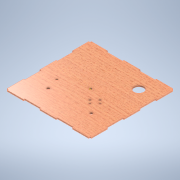
# Autodesk Inventor part: FloorPlateBottom_V2
Saved by Autodesk Inventor 2022.2 (Build 262287000, 287)
## iProperties
Created: 2022-11-22
Part Number: FloorPlateBottom_V2
Material: Wood (Oak)
Document SubType Name: Modeling
Designer: jaege
Density: 0.76 g/cm^3
Appearance: Red Oak - Natural Low Gloss
Mass: 194.404 g
Surface Area: 1333.29 cm^2
Volume: 255.795 cm^3
Author: jaege
Autodesk Inventor part; units mm, degrees
ref_plane "YZ Plane" through (0, 0, 0) normal (1, 0, 0) x (0, 1, 0)
ref_plane "XZ Plane" through (0, 0, 0) normal (0, 1, 0) x (-1, 0, 0)
ref_plane "XY Plane" through (0, 0, 0) normal (0, 0, 1) x (1, 0, 0)
sketch "Sketch1" plane through (0, 0, 0) normal (0, 1, 0) x (-1, 0, 0)
  line L0 (-125, 125) -> (125, 125)
  line L1 (125, 125) -> (125, -125)
  line L2 (125, -125) -> (-125, -125)
  line L3 (-125, -125) -> (-125, 125)
  line L4 (-125, 125) -> (125, -125) construction
  line L5 (125, 125) -> (-125, -125) construction
  line L6 (125, -125) -> (75, -125)
  line L7 (75, -125) -> (75, -129)
  line L8 (75, -129) -> (125, -129)
  line L9 (125, -129) -> (125, -125)
  line L10 (125, -125) -> (129, -125)
  line L11 (129, -125) -> (129, -75)
  line L12 (129, -75) -> (125, -75)
  line L13 (125, -75) -> (125, -125)
  line L14 (-125, -125) -> (-129, -125)
  line L15 (-129, -125) -> (-129, -75)
  line L16 (-129, -75) -> (-125, -75)
  line L17 (-125, -75) -> (-125, -125)
  line L18 (125, 125) -> (75, 125)
  line L19 (75, 125) -> (75, 129)
  line L20 (75, 129) -> (125, 129)
  line L21 (125, 129) -> (125, 125)
  line L22 (75, -129) -> (75, -125)
  line L23 (75, -125) -> (25, -125)
  line L24 (25, -125) -> (25, -129)
  line L25 (25, -129) -> (75, -129)
  line L26 (25, -129) -> (25, -125)
  line L27 (25, -125) -> (-25, -125)
  line L28 (-25, -125) -> (-25, -129)
  line L29 (-25, -129) -> (25, -129)
  line L30 (-25, -129) -> (-25, -125)
  line L31 (-25, -125) -> (-75, -125)
  line L32 (-75, -125) -> (-75, -129)
  line L33 (-75, -129) -> (-25, -129)
  line L34 (-75, -129) -> (-75, -125)
  line L35 (-75, -125) -> (-125, -125)
  line L36 (-125, -125) -> (-125, -129)
  line L37 (-125, -129) -> (-75, -129)
  line L38 (125, -75) -> (129, -75)
  line L39 (125, -25) -> (125, -75)
  line L40 (129, -25) -> (125, -25)
  line L41 (129, -75) -> (129, -25)
  line L42 (125, -25) -> (129, -25)
  line L43 (125, 25) -> (125, -25)
  line L44 (129, 25) -> (125, 25)
  line L45 (129, -25) -> (129, 25)
  line L46 (125, 25) -> (129, 25)
  line L47 (125, 75) -> (125, 25)
  line L48 (129, 75) -> (125, 75)
  line L49 (129, 25) -> (129, 75)
  line L50 (125, 75) -> (129, 75)
  line L51 (125, 125) -> (125, 75)
  line L52 (129, 125) -> (125, 125)
  line L53 (129, 75) -> (129, 125)
  line L54 (-125, -75) -> (-129, -75)
  line L55 (-129, -75) -> (-129, -25)
  line L56 (-129, -25) -> (-125, -25)
  line L57 (-125, -25) -> (-125, -75)
  line L58 (-125, -25) -> (-129, -25)
  line L59 (-129, -25) -> (-129, 25)
  line L60 (-129, 25) -> (-125, 25)
  line L61 (-125, 25) -> (-125, -25)
  line L62 (-125, 25) -> (-129, 25)
  line L63 (-129, 25) -> (-129, 75)
  line L64 (-129, 75) -> (-125, 75)
  line L65 (-125, 75) -> (-125, 25)
  line L66 (-125, 75) -> (-129, 75)
  line L67 (-129, 75) -> (-129, 125)
  line L68 (-129, 125) -> (-125, 125)
  line L69 (-125, 125) -> (-125, 75)
  line L70 (75, 125) -> (25, 125)
  line L71 (25, 125) -> (25, 129)
  line L72 (25, 129) -> (75, 129)
  line L73 (75, 129) -> (75, 125)
  line L74 (25, 125) -> (-25, 125)
  line L75 (-25, 125) -> (-25, 129)
  line L76 (-25, 129) -> (25, 129)
  line L77 (25, 129) -> (25, 125)
  line L78 (-25, 125) -> (-75, 125)
  line L79 (-75, 125) -> (-75, 129)
  line L80 (-75, 129) -> (-25, 129)
  line L81 (-25, 129) -> (-25, 125)
  line L82 (-75, 125) -> (-125, 125)
  line L83 (-125, 125) -> (-125, 129)
  line L84 (-125, 129) -> (-75, 129)
  line L85 (-75, 129) -> (-75, 125)
  point P0 (0, 0)
  dimension "d0" = 250
  dimension "d1" = 250
  dimension "d2" = 50
  dimension "d3" = 4
  dimension "d4" = 4
  dimension "d5" = 50
  dimension "d6" = 4
  dimension "d7" = 50
  dimension "d8" = 50
  dimension "d9" = 4
  dimension "d12" = 50
  dimension "d19" = 50
  dimension "d26" = 50
  dimension "d33" = 50
  constraints: 172 end point, 10 parallel, 7 horizontal, 5 perpendicular, 2 midpoint, 2 vertical, 136 other
  measures "d0" distance of L1.end L2.end
  measures "d1" distance of L0.end L1.end
  measures "d2" distance of L8.end L7.end
  measures "d3" distance of L7.end L6.end
  measures "d4" distance of L12.end L11.end
  measures "d5" distance of L11.end L10.end
  measures "d6" distance of L15.end L16.end
  measures "d7" distance of L14.end L15.end
  measures "d8" distance of L19.end L20.end
  measures "d9" distance of L18.end L19.end
  measures "d12" distance of L1.end L22.end
  measures "d19" distance of L1.end L38.start
  measures "d26" distance of L2.end L54.start
  measures "d33" distance of L0.end L70.start
extrude "Extrusion1" add sketch "Sketch1" along normal blind 4 contours L83 L84 L79 L0 | L0 L1 L2 L3 | L3 L64 L67 L68 | L75 L76 L71 L0 | L3 L56 L59 L60 | L19 L20 L21 L0 | L3 L14 L15 L16 | L52 L53 L48 L1 | L2 L32 L37 L36 | L44 L45 L40 L1 | L2 L24 L29 L28 | L12 L11 L10 L1 | L2 L9 L8 L7
sketch "Sketch2" plane through (0, 4, 0) normal (0, 1, 0) x (1, 0, 0)
  line L0 (25, -125) -> (75, -125) construction
  circle A0 centre (0, 2.3) radius 3.5
  line L1 (-8.45, 2.3) -> (8.45, 2.3) construction
  line L2 (-8.45, 1.0705) -> (8.45, 1.0705) construction
  line L3 (8.45, 3.5295) -> (-8.45, 3.5295) construction
  arc A1 (-8.45, 3.5295) -> (-8.45, 1.0705) centre (-8.45, 2.3) ccw construction
  arc A2 (8.45, 1.0705) -> (8.45, 3.5295) centre (8.45, 2.3) ccw construction
  circle A3 centre (8.45, 2.3) radius 1.2295
  circle A4 centre (-8.45, 2.3) radius 1.2295
  circle A5 centre (-66, -62.2) radius 4
  circle A6 centre (66, -62.2) radius 4
  line L4 (0, 180.6) -> (0, -180.6) construction
  line L5 (-93.2324, -124) -> (95.467, -124) construction
  line L6 (-129, -125) -> (-125, -125) projected
  line L7 (25, -29.4721) -> (29.2426, -25.2294)
  line L8 (44.799, -9.6731) -> (47.6274, -12.5015)
  line L9 (47.6274, -12.5015) -> (43.3848, -16.7442)
  line L10 (27.8284, -32.3005) -> (25, -29.4721)
  line L11 (34.8995, -39.3716) -> (39.1421, -35.1289)
  line L12 (54.6985, -19.5726) -> (57.5269, -22.401)
  line L13 (57.5269, -22.401) -> (53.2843, -26.6437)
  line L14 (37.7279, -42.2) -> (34.8995, -39.3716)
  line L15 (40.5563, -13.9157) -> (43.3848, -16.7442)
  line L16 (29.2426, -25.2294) -> (32.0711, -28.0579)
  line L17 (39.1421, -35.1289) -> (41.9706, -37.9574)
  line L18 (50.4558, -23.8152) -> (53.2843, -26.6437)
  line L19 (40.5563, -13.9157) -> (44.799, -9.6731)
  line L20 (29.2426, -25.2294) -> (40.5563, -13.9157) construction
  line L21 (43.3848, -16.7442) -> (32.0711, -28.0579) construction
  line L22 (50.4558, -23.8152) -> (54.6985, -19.5726)
  line L23 (53.2843, -26.6437) -> (41.9706, -37.9574) construction
  line L24 (32.0711, -28.0579) -> (27.8284, -32.3005)
  line L25 (39.1421, -35.1289) -> (50.4558, -23.8152) construction
  line L26 (41.9706, -37.9574) -> (37.7279, -42.2)
  point P0 (0, 0)
  point P1 (26.4142, -30.8863)
  dimension "d46" = 7
  dimension "d47" = 16.9
  dimension "d48" = 1.2295
  dimension "d52" = 8
  dimension "d53" = 132
  dimension "d54" = 61.8
  dimension "d55" = 1
  dimension "d56" = 64.5
  dimension "d57" = 10
  dimension "d58" = 4
  dimension "d59" = 6
  dimension "d60" = 6
  dimension "d61" = 45
  dimension "d62" = 20
  dimension "d63" = 28
  dimension "d64" = 25
  constraints: 50 end point, 21 parallel, 15 perpendicular, 7 centre point, 6 point on line, 4 point on circle, 4 tangent, 3 collinear, 3 equal radius, 2 coincident, 2 horizontal, 2 midpoint, 1 horizontal alignment, 1 symmetric about line, 1 vertical alignment
  measures "d46" diameter of A0
  measures "d47" distance of L1.start L1.end
  measures "d48" radius of A2
  measures "d52" diameter of A5
  measures "d53" distance of A6.centre A5.centre
  measures "d54" distance from line of A6.centre L5
  measures "d55" distance between parallel lines of L6 L5
  measures "d56" vertical distance of A5.centre A0.centre
  measures "d57" distance between parallel lines of L11 L9
  measures "d58" distance of L8.start L8.end
  measures "d59" distance of L8.start L15.start
  measures "d60" distance from line of point (26.414, -30.886) L16
  measures "d61" angle of L4 L7
  measures "d62" vertical distance of A6.centre L14.start
  measures "d63" distance of L12.end L14.start
  measures "d64" distance from line of L4 L7.start
extrude "Extrusion2" cut sketch "Sketch2" against normal up to next
sketch "Sketch3" plane through (0, 4, 0) normal (0, 1, 0) x (1, 0, 0)
  point P0 (0, 0)
sketch "Sketch4" plane through (0, 4, 0) normal (0, 1, 0) x (1, 0, 0)
  circle A0 centre (75, 75) radius 15
  line L0 (125, 25) -> (125, 75) projected
  line L1 (75, 125) -> (25, 125) projected
  point P0 (0, 0)
  dimension "d65" = 30
  dimension "d66" = 50
  dimension "d67" = 50
  constraints: 1 centre point
  measures "d65" diameter of A0
  measures "d66" distance from line of L0 A0.centre
  measures "d67" distance from line of L1 A0.centre
extrude "Extrusion3" cut sketch "Sketch4" against normal through all
sketch "Sketch5" plane through (0, 4, 0) normal (0, 1, 0) x (1, 0, 0)
  circle A0 centre (75, 75) radius 15 projected
  line L0 (54.6985, -19.5726) -> (57.5269, -22.401) projected
  line L1 (57.5269, -22.401) -> (53.2843, -26.6437) projected
  line L2 (53.2843, -26.6437) -> (50.4558, -23.8152) projected
  line L3 (50.4558, -23.8152) -> (54.6985, -19.5726) projected
  circle A1 centre (8.45, 2.3) radius 1.2295 projected
  circle A2 centre (0, 2.3) radius 3.5 projected
  line L4 (39.1421, -35.1289) -> (41.9706, -37.9574) projected
  line L5 (41.9706, -37.9574) -> (37.7279, -42.2) projected
  line L6 (37.7279, -42.2) -> (34.8995, -39.3716) projected
  line L7 (34.8995, -39.3716) -> (39.1421, -35.1289) projected
  line L8 (44.799, -9.6731) -> (47.6274, -12.5015) projected
  line L9 (47.6274, -12.5015) -> (43.3848, -16.7442) projected
  line L10 (43.3848, -16.7442) -> (40.5563, -13.9157) projected
  line L11 (40.5563, -13.9157) -> (44.799, -9.6731) projected
  circle A3 centre (66, -62.2) radius 4 projected
  circle A4 centre (-8.45, 2.3) radius 1.2295 projected
  circle A5 centre (-66, -62.2) radius 4 projected
  line L12 (29.2426, -25.2294) -> (32.0711, -28.0579) projected
  line L13 (32.0711, -28.0579) -> (27.8284, -32.3005) projected
  line L14 (27.8284, -32.3005) -> (25, -29.4721) projected
  line L15 (25, -29.4721) -> (29.2426, -25.2294) projected
  line L16 (-129, -125) -> (-125, -125) projected
  line L17 (-125, -125) -> (-125, -129) projected
  line L18 (-125, -129) -> (-75, -129) projected
  line L19 (-75, -129) -> (-75, -125) projected
  line L20 (-75, -125) -> (-25, -125) projected
  line L21 (-25, -125) -> (-25, -129) projected
  line L22 (-25, -129) -> (25, -129) projected
  line L23 (25, -129) -> (25, -125) projected
  line L24 (25, -125) -> (75, -125) projected
  line L25 (75, -125) -> (75, -129) projected
  line L26 (75, -129) -> (125, -129) projected
  line L27 (125, -129) -> (125, -125) projected
  line L28 (125, -125) -> (129, -125) projected
  line L29 (129, -125) -> (129, -75) projected
  line L30 (129, -75) -> (125, -75) projected
  line L31 (125, -75) -> (125, -25) projected
  line L32 (125, -25) -> (129, -25) projected
  line L33 (129, -25) -> (129, 25) projected
  line L34 (129, 25) -> (125, 25) projected
  line L35 (125, 25) -> (125, 75) projected
  line L36 (125, 75) -> (129, 75) projected
  line L37 (129, 75) -> (129, 125) projected
  line L38 (129, 125) -> (125, 125) projected
  line L39 (125, 125) -> (125, 129) projected
  line L40 (125, 129) -> (75, 129) projected
  line L41 (75, 129) -> (75, 125) projected
  line L42 (75, 125) -> (25, 125) projected
  line L43 (25, 125) -> (25, 129) projected
  line L44 (25, 129) -> (-25, 129) projected
  line L45 (-25, 129) -> (-25, 125) projected
  line L46 (-25, 125) -> (-75, 125) projected
  line L47 (-75, 125) -> (-75, 129) projected
  line L48 (-75, 129) -> (-125, 129) projected
  line L49 (-125, 129) -> (-125, 125) projected
  line L50 (-125, 125) -> (-129, 125) projected
  line L51 (-129, 125) -> (-129, 75) projected
  line L52 (-129, 75) -> (-125, 75) projected
  line L53 (-125, 75) -> (-125, 25) projected
  line L54 (-125, 25) -> (-129, 25) projected
  line L55 (-129, 25) -> (-129, -25) projected
  line L56 (-129, -25) -> (-125, -25) projected
  line L57 (-125, -25) -> (-125, -75) projected
  line L58 (-125, -75) -> (-129, -75) projected
  line L59 (-129, -75) -> (-129, -125) projected
  line L60 (-77.5858, -28.5858) -> (-73.3431, -24.3431)
  line L61 (-73.3431, -24.3431) -> (-76.1716, -21.5147)
  line L62 (-76.1716, -21.5147) -> (-80.4142, -25.7574)
  line L63 (-80.4142, -25.7574) -> (-77.5858, -28.5858)
  line L64 (-79, -30) -> (-71.9289, -22.9289) construction
  line L65 (-78.2929, -23.636) -> (-75.4645, -26.4645) construction
  point P0 (0, 0)
  dimension "d70" = 45
  dimension "d71" = 6
  dimension "d72" = 4
  dimension "d73" = 10
  dimension "d74" = 95
  dimension "d75" = 46
  constraints: 12 end point, 3 midpoint, 2 parallel, 1 collinear, 1 perpendicular
  measures "d70" angle of L20 L60
  measures "d71" distance of L61.end L62.end
  measures "d72" distance of L60.end L61.end
  measures "d73" distance of L64.start L64.end
  measures "d74" distance from line of L20 L64.start
  measures "d75" distance from line of L57 L64.start
extrude "Extrusion4" cut sketch "Sketch5" against normal through all contours L63 L62 L61 L60
body "Solid1"
